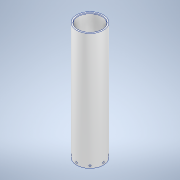
# Autodesk Inventor part: Combustion Chamber
Saved by Autodesk Inventor 2021 (Build 250183000, 183)
## iProperties
Created: 2021-02-14
Part Number: Combustion Chamber
Material: Aluminum 6061
Document SubType Name: Modeling
Designer: dscol
Density: 2.7 g/cm^3
Appearance: Aluminum - Flat
Mass: 2947.64 g
Surface Area: 3491.4 cm^2
Volume: 1091.72 cm^3
Author: dscol
Autodesk Inventor part; units mm, degrees
ref_plane "XZ Plane" through (0, 0, 0) normal (0, 1, 0) x (-1, 0, 0)
ref_plane "XY Plane" through (0, 0, 0) normal (0, 0, 1) x (1, 0, 0)
sketch "Sketch1" plane through (0, 0, 0) normal (0, 1, 0) x (-1, 0, 0)
  circle A0 centre (0, 0) radius 57.15
  dimension "d0" = 114.3
  constraints: 1 centre point, 1 coincident
  measures "d0" diameter of A0
extrude "Extrusion1" add sketch "Sketch1" along normal blind 498.475
sketch "Sketch2" plane through (0, 498.475, 0) normal (0, 1, 0) x (1, 0, 0)
  circle A0 centre (0, 0) radius 50.8
  dimension "d3" = 101.6
  constraints: 1 centre point, 1 coincident
  measures "d3" diameter of A0
extrude "Extrusion2" cut sketch "Sketch2" against normal blind 609.6
ref_plane "Work Plane1" through (57.15, 0, 0) normal (1, 0, 0) x (0, 1, 0)
chamfer "Chamfer1" distance 3.175 angle 15 1 edges at (-50.8, 498.475, 0) measured on face at (-13.148, 166.1583, 49.069)
sketch "Sketch4" plane through (0, 0, 0) normal (0, 0, 1) x (1, 0, 0)
  circle A0 centre (0, 10.16) radius 3.3782
  point P0 (0, 0)
  dimension "d21" = 10.16
  dimension "d22" = 6.7564
  constraints: 1 centre point, 1 vertical alignment
  measures "d21" distance of point (0, 0) A0.centre
  measures "d22" diameter of A0
extrude "Extrusion3" cut sketch "Sketch4" along normal through all
pattern_circular "Circular Pattern2" count 8 over 360 about axis through (0, -10, 0) along (0, 1, 0) of "Extrusion3"
chamfer "Chamfer2" distance 3.175 angle 15 1 edges at (-50.8, 0, 0) measured on face at (25.4, 165.1, 43.9941)
body "Solid1"
